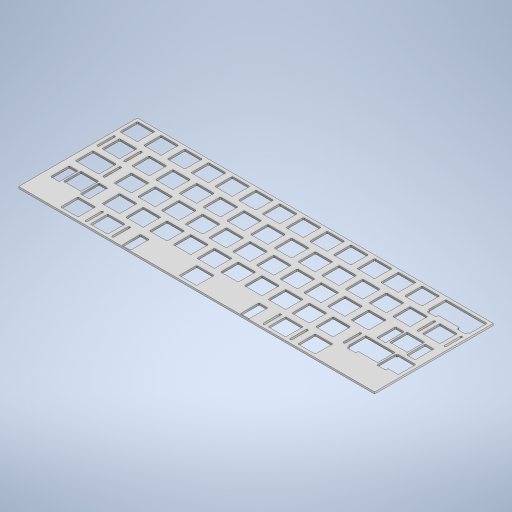
# Autodesk Inventor part: plate
Saved by Autodesk Inventor 2024.2 (Build 282272000, 272)
## iProperties
Created: 2024-07-29
Part Number: plate
Material: Generic
Document SubType Name: Modeling
Designer: Eric
Density: 1 g/cm^3
Appearance: Default
Author: Eric
Autodesk Inventor part; units mm, degrees
ref_plane "YZ Plane" through (0, 0, 0) normal (1, 0, 0) x (0, 1, 0)
ref_plane "XZ Plane" through (0, 0, 0) normal (0, 1, 0) x (-1, 0, 0)
ref_plane "XY Plane" through (0, 0, 0) normal (0, 0, 1) x (1, 0, 0)
sketch "Sketch1" plane through (0, 0, 0) normal (0, 1, 0) x (-1, 0, 0)
  line L0 (-3.025, 2.525) -> (-16.025, 2.525)
  line L1 (-3.025, 16.525) -> (-16.025, 16.525)
  line L2 (-2.525, 3.025) -> (-2.525, 16.025)
  line L3 (-16.525, 3.025) -> (-16.525, 16.025)
  arc A0 (-3.025, 2.525) -> (-2.525, 3.025) centre (-3.025, 3.025) ccw
  arc A1 (-16.525, 3.025) -> (-16.025, 2.525) centre (-16.025, 3.025) ccw
  arc A2 (-2.525, 16.025) -> (-3.025, 16.525) centre (-3.025, 16.025) ccw
  arc A3 (-16.025, 16.525) -> (-16.525, 16.025) centre (-16.025, 16.025) ccw
  line L4 (-22.075, 2.525) -> (-35.075, 2.525)
  line L5 (-22.075, 16.525) -> (-35.075, 16.525)
  line L6 (-21.575, 3.025) -> (-21.575, 16.025)
  line L7 (-35.575, 3.025) -> (-35.575, 16.025)
  arc A4 (-22.075, 2.525) -> (-21.575, 3.025) centre (-22.075, 3.025) ccw
  arc A5 (-35.575, 3.025) -> (-35.075, 2.525) centre (-35.075, 3.025) ccw
  arc A6 (-21.575, 16.025) -> (-22.075, 16.525) centre (-22.075, 16.025) ccw
  arc A7 (-35.075, 16.525) -> (-35.575, 16.025) centre (-35.075, 16.025) ccw
  line L8 (-41.125, 2.525) -> (-54.125, 2.525)
  line L9 (-41.125, 16.525) -> (-54.125, 16.525)
  line L10 (-40.625, 3.025) -> (-40.625, 16.025)
  line L11 (-54.625, 3.025) -> (-54.625, 16.025)
  arc A8 (-41.125, 2.525) -> (-40.625, 3.025) centre (-41.125, 3.025) ccw
  arc A9 (-54.625, 3.025) -> (-54.125, 2.525) centre (-54.125, 3.025) ccw
  arc A10 (-40.625, 16.025) -> (-41.125, 16.525) centre (-41.125, 16.025) ccw
  arc A11 (-54.125, 16.525) -> (-54.625, 16.025) centre (-54.125, 16.025) ccw
  line L12 (-60.175, 2.525) -> (-73.175, 2.525)
  line L13 (-60.175, 16.525) -> (-73.175, 16.525)
  line L14 (-59.675, 3.025) -> (-59.675, 16.025)
  line L15 (-73.675, 3.025) -> (-73.675, 16.025)
  arc A12 (-60.175, 2.525) -> (-59.675, 3.025) centre (-60.175, 3.025) ccw
  arc A13 (-73.675, 3.025) -> (-73.175, 2.525) centre (-73.175, 3.025) ccw
  arc A14 (-59.675, 16.025) -> (-60.175, 16.525) centre (-60.175, 16.025) ccw
  arc A15 (-73.175, 16.525) -> (-73.675, 16.025) centre (-73.175, 16.025) ccw
  line L16 (-79.225, 2.525) -> (-92.225, 2.525)
  line L17 (-79.225, 16.525) -> (-92.225, 16.525)
  line L18 (-78.725, 3.025) -> (-78.725, 16.025)
  line L19 (-92.725, 3.025) -> (-92.725, 16.025)
  arc A16 (-79.225, 2.525) -> (-78.725, 3.025) centre (-79.225, 3.025) ccw
  arc A17 (-92.725, 3.025) -> (-92.225, 2.525) centre (-92.225, 3.025) ccw
  arc A18 (-78.725, 16.025) -> (-79.225, 16.525) centre (-79.225, 16.025) ccw
  arc A19 (-92.225, 16.525) -> (-92.725, 16.025) centre (-92.225, 16.025) ccw
  line L20 (-98.275, 2.525) -> (-111.275, 2.525)
  line L21 (-98.275, 16.525) -> (-111.275, 16.525)
  line L22 (-97.775, 3.025) -> (-97.775, 16.025)
  line L23 (-111.775, 3.025) -> (-111.775, 16.025)
  arc A20 (-98.275, 2.525) -> (-97.775, 3.025) centre (-98.275, 3.025) ccw
  arc A21 (-111.775, 3.025) -> (-111.275, 2.525) centre (-111.275, 3.025) ccw
  arc A22 (-97.775, 16.025) -> (-98.275, 16.525) centre (-98.275, 16.025) ccw
  arc A23 (-111.275, 16.525) -> (-111.775, 16.025) centre (-111.275, 16.025) ccw
  line L24 (-117.325, 2.525) -> (-130.325, 2.525)
  line L25 (-117.325, 16.525) -> (-130.325, 16.525)
  line L26 (-116.825, 3.025) -> (-116.825, 16.025)
  line L27 (-130.825, 3.025) -> (-130.825, 16.025)
  arc A24 (-117.325, 2.525) -> (-116.825, 3.025) centre (-117.325, 3.025) ccw
  arc A25 (-130.825, 3.025) -> (-130.325, 2.525) centre (-130.325, 3.025) ccw
  arc A26 (-116.825, 16.025) -> (-117.325, 16.525) centre (-117.325, 16.025) ccw
  arc A27 (-130.325, 16.525) -> (-130.825, 16.025) centre (-130.325, 16.025) ccw
  line L28 (-136.375, 2.525) -> (-149.375, 2.525)
  line L29 (-136.375, 16.525) -> (-149.375, 16.525)
  line L30 (-135.875, 3.025) -> (-135.875, 16.025)
  line L31 (-149.875, 3.025) -> (-149.875, 16.025)
  arc A28 (-136.375, 2.525) -> (-135.875, 3.025) centre (-136.375, 3.025) ccw
  arc A29 (-149.875, 3.025) -> (-149.375, 2.525) centre (-149.375, 3.025) ccw
  arc A30 (-135.875, 16.025) -> (-136.375, 16.525) centre (-136.375, 16.025) ccw
  arc A31 (-149.375, 16.525) -> (-149.875, 16.025) centre (-149.375, 16.025) ccw
  line L32 (-155.425, 2.525) -> (-168.425, 2.525)
  line L33 (-155.425, 16.525) -> (-168.425, 16.525)
  line L34 (-154.925, 3.025) -> (-154.925, 16.025)
  line L35 (-168.925, 3.025) -> (-168.925, 16.025)
  arc A32 (-155.425, 2.525) -> (-154.925, 3.025) centre (-155.425, 3.025) ccw
  arc A33 (-168.925, 3.025) -> (-168.425, 2.525) centre (-168.425, 3.025) ccw
  arc A34 (-154.925, 16.025) -> (-155.425, 16.525) centre (-155.425, 16.025) ccw
  arc A35 (-168.425, 16.525) -> (-168.925, 16.025) centre (-168.425, 16.025) ccw
  line L36 (-174.475, 2.525) -> (-187.475, 2.525)
  line L37 (-174.475, 16.525) -> (-187.475, 16.525)
  line L38 (-173.975, 3.025) -> (-173.975, 16.025)
  line L39 (-187.975, 3.025) -> (-187.975, 16.025)
  arc A36 (-174.475, 2.525) -> (-173.975, 3.025) centre (-174.475, 3.025) ccw
  arc A37 (-187.975, 3.025) -> (-187.475, 2.525) centre (-187.475, 3.025) ccw
  arc A38 (-173.975, 16.025) -> (-174.475, 16.525) centre (-174.475, 16.025) ccw
  arc A39 (-187.475, 16.525) -> (-187.975, 16.025) centre (-187.475, 16.025) ccw
  line L40 (-193.525, 2.525) -> (-206.525, 2.525)
  line L41 (-193.525, 16.525) -> (-206.525, 16.525)
  line L42 (-193.025, 3.025) -> (-193.025, 16.025)
  line L43 (-207.025, 3.025) -> (-207.025, 16.025)
  arc A40 (-193.525, 2.525) -> (-193.025, 3.025) centre (-193.525, 3.025) ccw
  arc A41 (-207.025, 3.025) -> (-206.525, 2.525) centre (-206.525, 3.025) ccw
  arc A42 (-193.025, 16.025) -> (-193.525, 16.525) centre (-193.525, 16.025) ccw
  arc A43 (-206.525, 16.525) -> (-207.025, 16.025) centre (-206.525, 16.025) ccw
  line L44 (-212.575, 2.525) -> (-225.575, 2.525)
  line L45 (-212.575, 16.525) -> (-225.575, 16.525)
  line L46 (-212.075, 3.025) -> (-212.075, 16.025)
  line L47 (-226.075, 3.025) -> (-226.075, 16.025)
  arc A44 (-212.575, 2.525) -> (-212.075, 3.025) centre (-212.575, 3.025) ccw
  arc A45 (-226.075, 3.025) -> (-225.575, 2.525) centre (-225.575, 3.025) ccw
  arc A46 (-212.075, 16.025) -> (-212.575, 16.525) centre (-212.575, 16.025) ccw
  arc A47 (-225.575, 16.525) -> (-226.075, 16.025) centre (-225.575, 16.025) ccw
  line L48 (-231.625, 2.525) -> (-244.625, 2.525)
  line L49 (-231.625, 16.525) -> (-244.625, 16.525)
  line L50 (-231.125, 3.025) -> (-231.125, 16.025)
  line L51 (-245.125, 3.025) -> (-245.125, 16.025)
  arc A48 (-231.625, 2.525) -> (-231.125, 3.025) centre (-231.625, 3.025) ccw
  arc A49 (-245.125, 3.025) -> (-244.625, 2.525) centre (-244.625, 3.025) ccw
  arc A50 (-231.125, 16.025) -> (-231.625, 16.525) centre (-231.625, 16.025) ccw
  arc A51 (-244.625, 16.525) -> (-245.125, 16.025) centre (-244.625, 16.025) ccw
  line L52 (-260.2, 2.525) -> (-273.2, 2.525)
  line L53 (-260.2, 16.525) -> (-273.2, 16.525)
  line L54 (-251.762, 18.525) -> (-257.762, 18.525)
  line L55 (-251.262, 17.025) -> (-251.262, 18.025)
  line L56 (-258.262, 17.025) -> (-258.262, 18.025)
  arc A52 (-251.262, 18.025) -> (-251.762, 18.525) centre (-251.762, 18.025) ccw
  arc A53 (-257.762, 18.525) -> (-258.262, 18.025) centre (-257.762, 18.025) ccw
  line L57 (-275.638, 18.525) -> (-281.638, 18.525)
  line L58 (-275.138, 17.025) -> (-275.138, 18.025)
  line L59 (-282.138, 17.025) -> (-282.138, 18.025)
  arc A54 (-275.138, 18.025) -> (-275.638, 18.525) centre (-275.638, 18.025) ccw
  arc A55 (-281.638, 18.525) -> (-282.138, 18.025) centre (-281.638, 18.025) ccw
  line L60 (-250.675, 2.525) -> (-263.675, 2.525)
  line L61 (-250.175, 3.025) -> (-250.175, 16.025)
  arc A56 (-250.675, 2.525) -> (-250.175, 3.025) centre (-250.675, 3.025) ccw
  arc A57 (-250.175, 16.025) -> (-250.675, 16.525) centre (-250.675, 16.025) ccw
  line L62 (-269.725, 2.525) -> (-282.725, 2.525)
  line L63 (-283.225, 3.025) -> (-283.225, 16.025)
  arc A58 (-283.225, 3.025) -> (-282.725, 2.525) centre (-282.725, 3.025) ccw
  arc A59 (-282.725, 16.525) -> (-283.225, 16.025) centre (-282.725, 16.025) ccw
  line L64 (-7.7875, 21.575) -> (-20.7875, 21.575)
  line L65 (-7.7875, 35.575) -> (-20.7875, 35.575)
  line L66 (-7.2875, 22.075) -> (-7.2875, 35.075)
  line L67 (-21.2875, 22.075) -> (-21.2875, 35.075)
  arc A60 (-7.7875, 21.575) -> (-7.2875, 22.075) centre (-7.7875, 22.075) ccw
  arc A61 (-21.2875, 22.075) -> (-20.7875, 21.575) centre (-20.7875, 22.075) ccw
  arc A62 (-7.2875, 35.075) -> (-7.7875, 35.575) centre (-7.7875, 35.075) ccw
  arc A63 (-20.7875, 35.575) -> (-21.2875, 35.075) centre (-20.7875, 35.075) ccw
  line L68 (-3.2875, 21.575) -> (-3.7875, 21.575)
  line L69 (-3.2875, 35.575) -> (-3.7875, 35.575)
  line L70 (-2.7875, 22.075) -> (-2.7875, 35.075)
  line L71 (-4.2875, 22.075) -> (-4.2875, 35.075)
  arc A64 (-3.2875, 21.575) -> (-2.7875, 22.075) centre (-3.2875, 22.075) ccw
  arc A65 (-4.2875, 22.075) -> (-3.7875, 21.575) centre (-3.7875, 22.075) ccw
  arc A66 (-2.7875, 35.075) -> (-3.2875, 35.575) centre (-3.2875, 35.075) ccw
  arc A67 (-3.7875, 35.575) -> (-4.2875, 35.075) centre (-3.7875, 35.075) ccw
  line L72 (-24.7875, 21.575) -> (-25.2875, 21.575)
  line L73 (-24.7875, 35.575) -> (-25.2875, 35.575)
  line L74 (-24.2875, 22.075) -> (-24.2875, 35.075)
  line L75 (-25.7875, 22.075) -> (-25.7875, 35.075)
  arc A68 (-24.7875, 21.575) -> (-24.2875, 22.075) centre (-24.7875, 22.075) ccw
  arc A69 (-25.7875, 22.075) -> (-25.2875, 21.575) centre (-25.2875, 22.075) ccw
  arc A70 (-24.2875, 35.075) -> (-24.7875, 35.575) centre (-24.7875, 35.075) ccw
  arc A71 (-25.2875, 35.575) -> (-25.7875, 35.075) centre (-25.2875, 35.075) ccw
  line L76 (-31.6, 21.575) -> (-44.6, 21.575)
  line L77 (-31.6, 35.575) -> (-44.6, 35.575)
  line L78 (-31.1, 22.075) -> (-31.1, 35.075)
  line L79 (-45.1, 22.075) -> (-45.1, 35.075)
  arc A72 (-31.6, 21.575) -> (-31.1, 22.075) centre (-31.6, 22.075) ccw
  arc A73 (-45.1, 22.075) -> (-44.6, 21.575) centre (-44.6, 22.075) ccw
  arc A74 (-31.1, 35.075) -> (-31.6, 35.575) centre (-31.6, 35.075) ccw
  arc A75 (-44.6, 35.575) -> (-45.1, 35.075) centre (-44.6, 35.075) ccw
  line L80 (-50.65, 21.575) -> (-63.65, 21.575)
  line L81 (-50.65, 35.575) -> (-63.65, 35.575)
  line L82 (-50.15, 22.075) -> (-50.15, 35.075)
  line L83 (-64.15, 22.075) -> (-64.15, 35.075)
  arc A76 (-50.65, 21.575) -> (-50.15, 22.075) centre (-50.65, 22.075) ccw
  arc A77 (-64.15, 22.075) -> (-63.65, 21.575) centre (-63.65, 22.075) ccw
  arc A78 (-50.15, 35.075) -> (-50.65, 35.575) centre (-50.65, 35.075) ccw
  arc A79 (-63.65, 35.575) -> (-64.15, 35.075) centre (-63.65, 35.075) ccw
  line L84 (-69.7, 21.575) -> (-82.7, 21.575)
  line L85 (-69.7, 35.575) -> (-82.7, 35.575)
  line L86 (-69.2, 22.075) -> (-69.2, 35.075)
  line L87 (-83.2, 22.075) -> (-83.2, 35.075)
  arc A80 (-69.7, 21.575) -> (-69.2, 22.075) centre (-69.7, 22.075) ccw
  arc A81 (-83.2, 22.075) -> (-82.7, 21.575) centre (-82.7, 22.075) ccw
  arc A82 (-69.2, 35.075) -> (-69.7, 35.575) centre (-69.7, 35.075) ccw
  arc A83 (-82.7, 35.575) -> (-83.2, 35.075) centre (-82.7, 35.075) ccw
  line L88 (-88.75, 21.575) -> (-101.75, 21.575)
  line L89 (-88.75, 35.575) -> (-101.75, 35.575)
  line L90 (-88.25, 22.075) -> (-88.25, 35.075)
  line L91 (-102.25, 22.075) -> (-102.25, 35.075)
  arc A84 (-88.75, 21.575) -> (-88.25, 22.075) centre (-88.75, 22.075) ccw
  arc A85 (-102.25, 22.075) -> (-101.75, 21.575) centre (-101.75, 22.075) ccw
  arc A86 (-88.25, 35.075) -> (-88.75, 35.575) centre (-88.75, 35.075) ccw
  arc A87 (-101.75, 35.575) -> (-102.25, 35.075) centre (-101.75, 35.075) ccw
  line L92 (-107.8, 21.575) -> (-120.8, 21.575)
  line L93 (-107.8, 35.575) -> (-120.8, 35.575)
  line L94 (-107.3, 22.075) -> (-107.3, 35.075)
  line L95 (-121.3, 22.075) -> (-121.3, 35.075)
  arc A88 (-107.8, 21.575) -> (-107.3, 22.075) centre (-107.8, 22.075) ccw
  arc A89 (-121.3, 22.075) -> (-120.8, 21.575) centre (-120.8, 22.075) ccw
  arc A90 (-107.3, 35.075) -> (-107.8, 35.575) centre (-107.8, 35.075) ccw
  arc A91 (-120.8, 35.575) -> (-121.3, 35.075) centre (-120.8, 35.075) ccw
  line L96 (-126.85, 21.575) -> (-139.85, 21.575)
  line L97 (-126.85, 35.575) -> (-139.85, 35.575)
  line L98 (-126.35, 22.075) -> (-126.35, 35.075)
  line L99 (-140.35, 22.075) -> (-140.35, 35.075)
  arc A92 (-126.85, 21.575) -> (-126.35, 22.075) centre (-126.85, 22.075) ccw
  arc A93 (-140.35, 22.075) -> (-139.85, 21.575) centre (-139.85, 22.075) ccw
  arc A94 (-126.35, 35.075) -> (-126.85, 35.575) centre (-126.85, 35.075) ccw
  arc A95 (-139.85, 35.575) -> (-140.35, 35.075) centre (-139.85, 35.075) ccw
  line L100 (-145.9, 21.575) -> (-158.9, 21.575)
  line L101 (-145.9, 35.575) -> (-158.9, 35.575)
  line L102 (-145.4, 22.075) -> (-145.4, 35.075)
  line L103 (-159.4, 22.075) -> (-159.4, 35.075)
  arc A96 (-145.9, 21.575) -> (-145.4, 22.075) centre (-145.9, 22.075) ccw
  arc A97 (-159.4, 22.075) -> (-158.9, 21.575) centre (-158.9, 22.075) ccw
  arc A98 (-145.4, 35.075) -> (-145.9, 35.575) centre (-145.9, 35.075) ccw
  arc A99 (-158.9, 35.575) -> (-159.4, 35.075) centre (-158.9, 35.075) ccw
  line L104 (-164.95, 21.575) -> (-177.95, 21.575)
  line L105 (-164.95, 35.575) -> (-177.95, 35.575)
  line L106 (-164.45, 22.075) -> (-164.45, 35.075)
  line L107 (-178.45, 22.075) -> (-178.45, 35.075)
  arc A100 (-164.95, 21.575) -> (-164.45, 22.075) centre (-164.95, 22.075) ccw
  arc A101 (-178.45, 22.075) -> (-177.95, 21.575) centre (-177.95, 22.075) ccw
  arc A102 (-164.45, 35.075) -> (-164.95, 35.575) centre (-164.95, 35.075) ccw
  arc A103 (-177.95, 35.575) -> (-178.45, 35.075) centre (-177.95, 35.075) ccw
  line L108 (-184, 21.575) -> (-197, 21.575)
  line L109 (-184, 35.575) -> (-197, 35.575)
  line L110 (-183.5, 22.075) -> (-183.5, 35.075)
  line L111 (-197.5, 22.075) -> (-197.5, 35.075)
  arc A104 (-184, 21.575) -> (-183.5, 22.075) centre (-184, 22.075) ccw
  arc A105 (-197.5, 22.075) -> (-197, 21.575) centre (-197, 22.075) ccw
  arc A106 (-183.5, 35.075) -> (-184, 35.575) centre (-184, 35.075) ccw
  arc A107 (-197, 35.575) -> (-197.5, 35.075) centre (-197, 35.075) ccw
  line L112 (-203.05, 21.575) -> (-216.05, 21.575)
  line L113 (-203.05, 35.575) -> (-216.05, 35.575)
  line L114 (-202.55, 22.075) -> (-202.55, 35.075)
  line L115 (-216.55, 22.075) -> (-216.55, 35.075)
  arc A108 (-203.05, 21.575) -> (-202.55, 22.075) centre (-203.05, 22.075) ccw
  arc A109 (-216.55, 22.075) -> (-216.05, 21.575) centre (-216.05, 22.075) ccw
  arc A110 (-202.55, 35.075) -> (-203.05, 35.575) centre (-203.05, 35.075) ccw
  arc A111 (-216.05, 35.575) -> (-216.55, 35.075) centre (-216.05, 35.075) ccw
  line L116 (-222.1, 21.575) -> (-235.1, 21.575)
  line L117 (-222.1, 35.575) -> (-235.1, 35.575)
  line L118 (-221.6, 22.075) -> (-221.6, 35.075)
  line L119 (-235.6, 22.075) -> (-235.6, 35.075)
  arc A112 (-222.1, 21.575) -> (-221.6, 22.075) centre (-222.1, 22.075) ccw
  arc A113 (-235.6, 22.075) -> (-235.1, 21.575) centre (-235.1, 22.075) ccw
  arc A114 (-221.6, 35.075) -> (-222.1, 35.575) centre (-222.1, 35.075) ccw
  arc A115 (-235.1, 35.575) -> (-235.6, 35.075) centre (-235.1, 35.075) ccw
  line L120 (-241.15, 21.575) -> (-254.15, 21.575)
  line L121 (-241.15, 35.575) -> (-254.15, 35.575)
  line L122 (-240.65, 22.075) -> (-240.65, 35.075)
  line L123 (-254.65, 22.075) -> (-254.65, 35.075)
  arc A116 (-241.15, 21.575) -> (-240.65, 22.075) centre (-241.15, 22.075) ccw
  arc A117 (-254.65, 22.075) -> (-254.15, 21.575) centre (-254.15, 22.075) ccw
  arc A118 (-240.65, 35.075) -> (-241.15, 35.575) centre (-241.15, 35.075) ccw
  arc A119 (-254.15, 35.575) -> (-254.65, 35.075) centre (-254.15, 35.075) ccw
  line L124 (-264.9625, 21.575) -> (-277.9625, 21.575)
  line L125 (-264.9625, 35.575) -> (-277.9625, 35.575)
  line L126 (-264.4625, 22.075) -> (-264.4625, 35.075)
  line L127 (-278.4625, 22.075) -> (-278.4625, 35.075)
  arc A120 (-264.9625, 21.575) -> (-264.4625, 22.075) centre (-264.9625, 22.075) ccw
  arc A121 (-278.4625, 22.075) -> (-277.9625, 21.575) centre (-277.9625, 22.075) ccw
  arc A122 (-264.4625, 35.075) -> (-264.9625, 35.575) centre (-264.9625, 35.075) ccw
  arc A123 (-277.9625, 35.575) -> (-278.4625, 35.075) centre (-277.9625, 35.075) ccw
  line L128 (-260.4625, 21.575) -> (-260.9625, 21.575)
  line L129 (-260.4625, 35.575) -> (-260.9625, 35.575)
  line L130 (-259.9625, 22.075) -> (-259.9625, 35.075)
  line L131 (-261.4625, 22.075) -> (-261.4625, 35.075)
  arc A124 (-260.4625, 21.575) -> (-259.9625, 22.075) centre (-260.4625, 22.075) ccw
  arc A125 (-261.4625, 22.075) -> (-260.9625, 21.575) centre (-260.9625, 22.075) ccw
  arc A126 (-259.9625, 35.075) -> (-260.4625, 35.575) centre (-260.4625, 35.075) ccw
  arc A127 (-260.9625, 35.575) -> (-261.4625, 35.075) centre (-260.9625, 35.075) ccw
  line L132 (-281.9625, 21.575) -> (-282.4625, 21.575)
  line L133 (-281.9625, 35.575) -> (-282.4625, 35.575)
  line L134 (-281.4625, 22.075) -> (-281.4625, 35.075)
  line L135 (-282.9625, 22.075) -> (-282.9625, 35.075)
  arc A128 (-281.9625, 21.575) -> (-281.4625, 22.075) centre (-281.9625, 22.075) ccw
  arc A129 (-282.9625, 22.075) -> (-282.4625, 21.575) centre (-282.4625, 22.075) ccw
  arc A130 (-281.4625, 35.075) -> (-281.9625, 35.575) centre (-281.9625, 35.075) ccw
  arc A131 (-282.4625, 35.575) -> (-282.9625, 35.075) centre (-282.4625, 35.075) ccw
  line L136 (-10.1687, 40.625) -> (-23.1687, 40.625)
  line L137 (-10.1687, 54.625) -> (-23.1687, 54.625)
  line L138 (-23.6687, 41.125) -> (-23.6687, 54.125)
  arc A132 (-23.6687, 41.125) -> (-23.1687, 40.625) centre (-23.1687, 41.125) ccw
  arc A133 (-23.1687, 54.625) -> (-23.6687, 54.125) centre (-23.1687, 54.125) ccw
  line L139 (-5.6687, 40.625) -> (-6.1687, 40.625)
  line L140 (-5.6687, 54.625) -> (-6.1687, 54.625)
  line L141 (-27.1687, 40.625) -> (-27.6687, 40.625)
  line L142 (-27.1687, 54.625) -> (-27.6687, 54.625)
  line L143 (-26.6687, 41.125) -> (-26.6687, 54.125)
  line L144 (-28.1687, 41.125) -> (-28.1687, 54.125)
  arc A134 (-27.1687, 40.625) -> (-26.6687, 41.125) centre (-27.1687, 41.125) ccw
  arc A135 (-28.1687, 41.125) -> (-27.6687, 40.625) centre (-27.6687, 41.125) ccw
  arc A136 (-26.6688, 54.125) -> (-27.1687, 54.625) centre (-27.1687, 54.125) ccw
  arc A137 (-27.6687, 54.625) -> (-28.1687, 54.125) centre (-27.6688, 54.125) ccw
  line L145 (-5.4062, 40.625) -> (-18.4062, 40.625)
  line L146 (-5.4062, 54.625) -> (-18.4062, 54.625)
  line L147 (-4.9062, 41.125) -> (-4.9062, 54.125)
  arc A138 (-5.4062, 40.625) -> (-4.9062, 41.125) centre (-5.4062, 41.125) ccw
  arc A139 (-4.9062, 54.125) -> (-5.4062, 54.625) centre (-5.4062, 54.125) ccw
  line L148 (-36.3625, 40.625) -> (-49.3625, 40.625)
  line L149 (-36.3625, 54.625) -> (-49.3625, 54.625)
  line L150 (-35.8625, 41.125) -> (-35.8625, 54.125)
  line L151 (-49.8625, 41.125) -> (-49.8625, 54.125)
  arc A140 (-36.3625, 40.625) -> (-35.8625, 41.125) centre (-36.3625, 41.125) ccw
  arc A141 (-49.8625, 41.125) -> (-49.3625, 40.625) centre (-49.3625, 41.125) ccw
  arc A142 (-35.8625, 54.125) -> (-36.3625, 54.625) centre (-36.3625, 54.125) ccw
  arc A143 (-49.3625, 54.625) -> (-49.8625, 54.125) centre (-49.3625, 54.125) ccw
  line L152 (-55.4125, 40.625) -> (-68.4125, 40.625)
  line L153 (-55.4125, 54.625) -> (-68.4125, 54.625)
  line L154 (-54.9125, 41.125) -> (-54.9125, 54.125)
  line L155 (-68.9125, 41.125) -> (-68.9125, 54.125)
  arc A144 (-55.4125, 40.625) -> (-54.9125, 41.125) centre (-55.4125, 41.125) ccw
  arc A145 (-68.9125, 41.125) -> (-68.4125, 40.625) centre (-68.4125, 41.125) ccw
  arc A146 (-54.9125, 54.125) -> (-55.4125, 54.625) centre (-55.4125, 54.125) ccw
  arc A147 (-68.4125, 54.625) -> (-68.9125, 54.125) centre (-68.4125, 54.125) ccw
  line L156 (-74.4625, 40.625) -> (-87.4625, 40.625)
  line L157 (-74.4625, 54.625) -> (-87.4625, 54.625)
  line L158 (-73.9625, 41.125) -> (-73.9625, 54.125)
  line L159 (-87.9625, 41.125) -> (-87.9625, 54.125)
  arc A148 (-74.4625, 40.625) -> (-73.9625, 41.125) centre (-74.4625, 41.125) ccw
  arc A149 (-87.9625, 41.125) -> (-87.4625, 40.625) centre (-87.4625, 41.125) ccw
  arc A150 (-73.9625, 54.125) -> (-74.4625, 54.625) centre (-74.4625, 54.125) ccw
  arc A151 (-87.4625, 54.625) -> (-87.9625, 54.125) centre (-87.4625, 54.125) ccw
  line L160 (-93.5125, 40.625) -> (-106.5125, 40.625)
  line L161 (-93.5125, 54.625) -> (-106.5125, 54.625)
  line L162 (-93.0125, 41.125) -> (-93.0125, 54.125)
  line L163 (-107.0125, 41.125) -> (-107.0125, 54.125)
  arc A152 (-93.5125, 40.625) -> (-93.0125, 41.125) centre (-93.5125, 41.125) ccw
  arc A153 (-107.0125, 41.125) -> (-106.5125, 40.625) centre (-106.5125, 41.125) ccw
  arc A154 (-93.0125, 54.125) -> (-93.5125, 54.625) centre (-93.5125, 54.125) ccw
  arc A155 (-106.5125, 54.625) -> (-107.0125, 54.125) centre (-106.5125, 54.125) ccw
  line L164 (-112.5625, 40.625) -> (-125.5625, 40.625)
  line L165 (-112.5625, 54.625) -> (-125.5625, 54.625)
  line L166 (-112.0625, 41.125) -> (-112.0625, 54.125)
  line L167 (-126.0625, 41.125) -> (-126.0625, 54.125)
  arc A156 (-112.5625, 40.625) -> (-112.0625, 41.125) centre (-112.5625, 41.125) ccw
  arc A157 (-126.0625, 41.125) -> (-125.5625, 40.625) centre (-125.5625, 41.125) ccw
  arc A158 (-112.0625, 54.125) -> (-112.5625, 54.625) centre (-112.5625, 54.125) ccw
  arc A159 (-125.5625, 54.625) -> (-126.0625, 54.125) centre (-125.5625, 54.125) ccw
  line L168 (-131.6125, 40.625) -> (-144.6125, 40.625)
  line L169 (-131.6125, 54.625) -> (-144.6125, 54.625)
  line L170 (-131.1125, 41.125) -> (-131.1125, 54.125)
  line L171 (-145.1125, 41.125) -> (-145.1125, 54.125)
  arc A160 (-131.6125, 40.625) -> (-131.1125, 41.125) centre (-131.6125, 41.125) ccw
  arc A161 (-145.1125, 41.125) -> (-144.6125, 40.625) centre (-144.6125, 41.125) ccw
  arc A162 (-131.1125, 54.125) -> (-131.6125, 54.625) centre (-131.6125, 54.125) ccw
  arc A163 (-144.6125, 54.625) -> (-145.1125, 54.125) centre (-144.6125, 54.125) ccw
  line L172 (-150.6625, 40.625) -> (-163.6625, 40.625)
  line L173 (-150.6625, 54.625) -> (-163.6625, 54.625)
  line L174 (-150.1625, 41.125) -> (-150.1625, 54.125)
  line L175 (-164.1625, 41.125) -> (-164.1625, 54.125)
  arc A164 (-150.6625, 40.625) -> (-150.1625, 41.125) centre (-150.6625, 41.125) ccw
  arc A165 (-164.1625, 41.125) -> (-163.6625, 40.625) centre (-163.6625, 41.125) ccw
  arc A166 (-150.1625, 54.125) -> (-150.6625, 54.625) centre (-150.6625, 54.125) ccw
  arc A167 (-163.6625, 54.625) -> (-164.1625, 54.125) centre (-163.6625, 54.125) ccw
  line L176 (-169.7125, 40.625) -> (-182.7125, 40.625)
  line L177 (-169.7125, 54.625) -> (-182.7125, 54.625)
  line L178 (-169.2125, 41.125) -> (-169.2125, 54.125)
  line L179 (-183.2125, 41.125) -> (-183.2125, 54.125)
  arc A168 (-169.7125, 40.625) -> (-169.2125, 41.125) centre (-169.7125, 41.125) ccw
  arc A169 (-183.2125, 41.125) -> (-182.7125, 40.625) centre (-182.7125, 41.125) ccw
  arc A170 (-169.2125, 54.125) -> (-169.7125, 54.625) centre (-169.7125, 54.125) ccw
  arc A171 (-182.7125, 54.625) -> (-183.2125, 54.125) centre (-182.7125, 54.125) ccw
  line L180 (-188.7625, 40.625) -> (-201.7625, 40.625)
  line L181 (-188.7625, 54.625) -> (-201.7625, 54.625)
  line L182 (-188.2625, 41.125) -> (-188.2625, 54.125)
  line L183 (-202.2625, 41.125) -> (-202.2625, 54.125)
  arc A172 (-188.7625, 40.625) -> (-188.2625, 41.125) centre (-188.7625, 41.125) ccw
  arc A173 (-202.2625, 41.125) -> (-201.7625, 40.625) centre (-201.7625, 41.125) ccw
  arc A174 (-188.2625, 54.125) -> (-188.7625, 54.625) centre (-188.7625, 54.125) ccw
  arc A175 (-201.7625, 54.625) -> (-202.2625, 54.125) centre (-201.7625, 54.125) ccw
  line L184 (-207.8125, 40.625) -> (-220.8125, 40.625)
  line L185 (-207.8125, 54.625) -> (-220.8125, 54.625)
  line L186 (-207.3125, 41.125) -> (-207.3125, 54.125)
  line L187 (-221.3125, 41.125) -> (-221.3125, 54.125)
  arc A176 (-207.8125, 40.625) -> (-207.3125, 41.125) centre (-207.8125, 41.125) ccw
  arc A177 (-221.3125, 41.125) -> (-220.8125, 40.625) centre (-220.8125, 41.125) ccw
  arc A178 (-207.3125, 54.125) -> (-207.8125, 54.625) centre (-207.8125, 54.125) ccw
  arc A179 (-220.8125, 54.625) -> (-221.3125, 54.125) centre (-220.8125, 54.125) ccw
  line L188 (-226.8625, 40.625) -> (-239.8625, 40.625)
  line L189 (-226.8625, 54.625) -> (-239.8625, 54.625)
  line L190 (-226.3625, 41.125) -> (-226.3625, 54.125)
  line L191 (-240.3625, 41.125) -> (-240.3625, 54.125)
  arc A180 (-226.8625, 40.625) -> (-226.3625, 41.125) centre (-226.8625, 41.125) ccw
  arc A181 (-240.3625, 41.125) -> (-239.8625, 40.625) centre (-239.8625, 41.125) ccw
  arc A182 (-226.3625, 54.125) -> (-226.8625, 54.625) centre (-226.8625, 54.125) ccw
  arc A183 (-239.8625, 54.625) -> (-240.3625, 54.125) centre (-239.8625, 54.125) ccw
  line L192 (-257.8188, 40.625) -> (-270.8188, 40.625)
  line L193 (-257.8188, 54.625) -> (-270.8188, 54.625)
  line L194 (-257.3188, 41.125) -> (-257.3187, 54.125)
  line L195 (-271.3188, 41.125) -> (-271.3188, 54.125)
  arc A184 (-257.8188, 40.625) -> (-257.3188, 41.125) centre (-257.8188, 41.125) ccw
  arc A185 (-271.3188, 41.125) -> (-270.8188, 40.625) centre (-270.8188, 41.125) ccw
  arc A186 (-257.3187, 54.125) -> (-257.8188, 54.625) centre (-257.8188, 54.125) ccw
  arc A187 (-270.8188, 54.625) -> (-271.3187, 54.125) centre (-270.8188, 54.125) ccw
  line L196 (-249.3808, 41.625) -> (-255.3808, 41.625)
  line L197 (-249.3807, 56.625) -> (-255.3807, 56.625)
  line L198 (-248.8808, 42.125) -> (-248.8808, 56.125)
  line L199 (-255.8808, 42.125) -> (-255.8808, 56.125)
  arc A188 (-249.3808, 41.625) -> (-248.8808, 42.125) centre (-249.3808, 42.125) ccw
  arc A189 (-255.8807, 42.125) -> (-255.3808, 41.625) centre (-255.3807, 42.125) ccw
  arc A190 (-248.8808, 56.125) -> (-249.3807, 56.625) centre (-249.3808, 56.125) ccw
  arc A191 (-255.3807, 56.625) -> (-255.8808, 56.125) centre (-255.3808, 56.125) ccw
  line L200 (-273.2568, 41.625) -> (-279.2568, 41.625)
  line L201 (-273.2568, 56.625) -> (-279.2568, 56.625)
  line L202 (-272.7568, 42.125) -> (-272.7568, 56.125)
  line L203 (-279.7568, 42.125) -> (-279.7568, 56.125)
  arc A192 (-273.2568, 41.625) -> (-272.7568, 42.125) centre (-273.2568, 42.125) ccw
  arc A193 (-279.7568, 42.125) -> (-279.2568, 41.625) centre (-279.2568, 42.125) ccw
  arc A194 (-272.7568, 56.125) -> (-273.2568, 56.625) centre (-273.2567, 56.125) ccw
  arc A195 (-279.2568, 56.625) -> (-279.7568, 56.125) centre (-279.2568, 56.125) ccw
  line L204 (-14.9312, 59.675) -> (-27.9312, 59.675)
  line L205 (-14.9312, 73.675) -> (-27.9312, 73.675)
  line L206 (-14.4312, 60.175) -> (-14.4312, 73.175)
  line L207 (-28.4312, 60.175) -> (-28.4313, 73.175)
  arc A196 (-14.9312, 59.675) -> (-14.4312, 60.175) centre (-14.9312, 60.175) ccw
  arc A197 (-28.4312, 60.175) -> (-27.9312, 59.675) centre (-27.9312, 60.175) ccw
  arc A198 (-14.4312, 73.175) -> (-14.9312, 73.675) centre (-14.9312, 73.175) ccw
  arc A199 (-27.9312, 73.675) -> (-28.4312, 73.175) centre (-27.9312, 73.175) ccw
  line L208 (-6.4932, 60.675) -> (-12.4932, 60.675)
  line L209 (-6.4932, 75.675) -> (-12.4932, 75.675)
  line L210 (-5.9932, 61.175) -> (-5.9932, 75.175)
  line L211 (-12.9932, 61.175) -> (-12.9932, 75.175)
  arc A200 (-6.4932, 60.675) -> (-5.9932, 61.175) centre (-6.4932, 61.175) ccw
  arc A201 (-12.9932, 61.175) -> (-12.4932, 60.675) centre (-12.4932, 61.175) ccw
  arc A202 (-5.9932, 75.175) -> (-6.4932, 75.675) centre (-6.4932, 75.175) ccw
  arc A203 (-12.4932, 75.675) -> (-12.9932, 75.175) centre (-12.4932, 75.175) ccw
  line L212 (-30.3692, 60.675) -> (-36.3692, 60.675)
  line L213 (-30.3692, 75.675) -> (-36.3692, 75.675)
  line L214 (-29.8693, 61.175) -> (-29.8692, 75.175)
  line L215 (-36.8692, 61.175) -> (-36.8693, 75.175)
  arc A204 (-30.3692, 60.675) -> (-29.8693, 61.175) centre (-30.3693, 61.175) ccw
  arc A205 (-36.8692, 61.175) -> (-36.3692, 60.675) centre (-36.3692, 61.175) ccw
  arc A206 (-29.8692, 75.175) -> (-30.3692, 75.675) centre (-30.3692, 75.175) ccw
  arc A207 (-36.3692, 75.675) -> (-36.8693, 75.175) centre (-36.3693, 75.175) ccw
  line L216 (-45.8875, 59.675) -> (-58.8875, 59.675)
  line L217 (-45.8875, 73.675) -> (-58.8875, 73.675)
  line L218 (-45.3875, 60.175) -> (-45.3875, 73.175)
  line L219 (-59.3875, 60.175) -> (-59.3875, 73.175)
  arc A208 (-45.8875, 59.675) -> (-45.3875, 60.175) centre (-45.8875, 60.175) ccw
  arc A209 (-59.3875, 60.175) -> (-58.8875, 59.675) centre (-58.8875, 60.175) ccw
  arc A210 (-45.3875, 73.175) -> (-45.8875, 73.675) centre (-45.8875, 73.175) ccw
  arc A211 (-58.8875, 73.675) -> (-59.3875, 73.175) centre (-58.8875, 73.175) ccw
  line L220 (-64.9375, 59.675) -> (-77.9375, 59.675)
  line L221 (-64.9375, 73.675) -> (-77.9375, 73.675)
  line L222 (-64.4375, 60.175) -> (-64.4375, 73.175)
  line L223 (-78.4375, 60.175) -> (-78.4375, 73.175)
  arc A212 (-64.9375, 59.675) -> (-64.4375, 60.175) centre (-64.9375, 60.175) ccw
  arc A213 (-78.4375, 60.175) -> (-77.9375, 59.675) centre (-77.9375, 60.175) ccw
  arc A214 (-64.4375, 73.175) -> (-64.9375, 73.675) centre (-64.9375, 73.175) ccw
  arc A215 (-77.9375, 73.675) -> (-78.4375, 73.175) centre (-77.9375, 73.175) ccw
  line L224 (-83.9875, 59.675) -> (-96.9875, 59.675)
  line L225 (-83.9875, 73.675) -> (-96.9875, 73.675)
  line L226 (-83.4875, 60.175) -> (-83.4875, 73.175)
  line L227 (-97.4875, 60.175) -> (-97.4875, 73.175)
  arc A216 (-83.9875, 59.675) -> (-83.4875, 60.175) centre (-83.9875, 60.175) ccw
  arc A217 (-97.4875, 60.175) -> (-96.9875, 59.675) centre (-96.9875, 60.175) ccw
  arc A218 (-83.4875, 73.175) -> (-83.9875, 73.675) centre (-83.9875, 73.175) ccw
  arc A219 (-96.9875, 73.675) -> (-97.4875, 73.175) centre (-96.9875, 73.175) ccw
  line L228 (-103.0375, 59.675) -> (-116.0375, 59.675)
  line L229 (-103.0375, 73.675) -> (-116.0375, 73.675)
  line L230 (-102.5375, 60.175) -> (-102.5375, 73.175)
  line L231 (-116.5375, 60.175) -> (-116.5375, 73.175)
  arc A220 (-103.0375, 59.675) -> (-102.5375, 60.175) centre (-103.0375, 60.175) ccw
  arc A221 (-116.5375, 60.175) -> (-116.0375, 59.675) centre (-116.0375, 60.175) ccw
  arc A222 (-102.5375, 73.175) -> (-103.0375, 73.675) centre (-103.0375, 73.175) ccw
  arc A223 (-116.0375, 73.675) -> (-116.5375, 73.175) centre (-116.0375, 73.175) ccw
  line L232 (-122.0875, 59.675) -> (-135.0875, 59.675)
  line L233 (-122.0875, 73.675) -> (-135.0875, 73.675)
  line L234 (-121.5875, 60.175) -> (-121.5875, 73.175)
  line L235 (-135.5875, 60.175) -> (-135.5875, 73.175)
  arc A224 (-122.0875, 59.675) -> (-121.5875, 60.175) centre (-122.0875, 60.175) ccw
  arc A225 (-135.5875, 60.175) -> (-135.0875, 59.675) centre (-135.0875, 60.175) ccw
  arc A226 (-121.5875, 73.175) -> (-122.0875, 73.675) centre (-122.0875, 73.175) ccw
  arc A227 (-135.0875, 73.675) -> (-135.5875, 73.175) centre (-135.0875, 73.175) ccw
  line L236 (-141.1375, 59.675) -> (-154.1375, 59.675)
  line L237 (-141.1375, 73.675) -> (-154.1375, 73.675)
  line L238 (-140.6375, 60.175) -> (-140.6375, 73.175)
  line L239 (-154.6375, 60.175) -> (-154.6375, 73.175)
  arc A228 (-141.1375, 59.675) -> (-140.6375, 60.175) centre (-141.1375, 60.175) ccw
  arc A229 (-154.6375, 60.175) -> (-154.1375, 59.675) centre (-154.1375, 60.175) ccw
  arc A230 (-140.6375, 73.175) -> (-141.1375, 73.675) centre (-141.1375, 73.175) ccw
  arc A231 (-154.1375, 73.675) -> (-154.6375, 73.175) centre (-154.1375, 73.175) ccw
  line L240 (-160.1875, 59.675) -> (-173.1875, 59.675)
  line L241 (-160.1875, 73.675) -> (-173.1875, 73.675)
  line L242 (-159.6875, 60.175) -> (-159.6875, 73.175)
  line L243 (-173.6875, 60.175) -> (-173.6875, 73.175)
  arc A232 (-160.1875, 59.675) -> (-159.6875, 60.175) centre (-160.1875, 60.175) ccw
  arc A233 (-173.6875, 60.175) -> (-173.1875, 59.675) centre (-173.1875, 60.175) ccw
  arc A234 (-159.6875, 73.175) -> (-160.1875, 73.675) centre (-160.1875, 73.175) ccw
  arc A235 (-173.1875, 73.675) -> (-173.6875, 73.175) centre (-173.1875, 73.175) ccw
  line L244 (-179.2375, 59.675) -> (-192.2375, 59.675)
  line L245 (-179.2375, 73.675) -> (-192.2375, 73.675)
  line L246 (-178.7375, 60.175) -> (-178.7375, 73.175)
  line L247 (-192.7375, 60.175) -> (-192.7375, 73.175)
  arc A236 (-179.2375, 59.675) -> (-178.7375, 60.175) centre (-179.2375, 60.175) ccw
  arc A237 (-192.7375, 60.175) -> (-192.2375, 59.675) centre (-192.2375, 60.175) ccw
  arc A238 (-178.7375, 73.175) -> (-179.2375, 73.675) centre (-179.2375, 73.175) ccw
  arc A239 (-192.2375, 73.675) -> (-192.7375, 73.175) centre (-192.2375, 73.175) ccw
  line L248 (-198.2875, 59.675) -> (-211.2875, 59.675)
  line L249 (-198.2875, 73.675) -> (-211.2875, 73.675)
  line L250 (-197.7875, 60.175) -> (-197.7875, 73.175)
  line L251 (-211.7875, 60.175) -> (-211.7875, 73.175)
  arc A240 (-198.2875, 59.675) -> (-197.7875, 60.175) centre (-198.2875, 60.175) ccw
  arc A241 (-211.7875, 60.175) -> (-211.2875, 59.675) centre (-211.2875, 60.175) ccw
  arc A242 (-197.7875, 73.175) -> (-198.2875, 73.675) centre (-198.2875, 73.175) ccw
  arc A243 (-211.2875, 73.675) -> (-211.7875, 73.175) centre (-211.2875, 73.175) ccw
  line L252 (-217.3375, 59.675) -> (-230.3375, 59.675)
  line L253 (-217.3375, 73.675) -> (-230.3375, 73.675)
  line L254 (-216.8375, 60.175) -> (-216.8375, 73.175)
  line L255 (-230.8375, 60.175) -> (-230.8375, 73.175)
  arc A244 (-217.3375, 59.675) -> (-216.8375, 60.175) centre (-217.3375, 60.175) ccw
  arc A245 (-230.8375, 60.175) -> (-230.3375, 59.675) centre (-230.3375, 60.175) ccw
  arc A246 (-216.8375, 73.175) -> (-217.3375, 73.675) centre (-217.3375, 73.175) ccw
  arc A247 (-230.3375, 73.675) -> (-230.8375, 73.175) centre (-230.3375, 73.175) ccw
  line L256 (-253.0563, 59.675) -> (-266.0563, 59.675)
  line L257 (-253.0563, 73.675) -> (-266.0562, 73.675)
  line L258 (-266.5562, 60.175) -> (-266.5562, 73.175)
  arc A248 (-266.5562, 60.175) -> (-266.0563, 59.675) centre (-266.0563, 60.175) ccw
  arc A249 (-266.0562, 73.675) -> (-266.5562, 73.175) centre (-266.0562, 73.175) ccw
  line L259 (-244.6183, 75.675) -> (-250.6182, 75.675)
  line L260 (-244.1182, 74.175) -> (-244.1182, 75.175)
  line L261 (-251.1182, 74.175) -> (-251.1182, 75.175)
  arc A250 (-244.1182, 75.175) -> (-244.6183, 75.675) centre (-244.6183, 75.175) ccw
  arc A251 (-250.6182, 75.675) -> (-251.1182, 75.175) centre (-250.6182, 75.175) ccw
  line L262 (-268.4943, 60.675) -> (-268.725, 60.675)
  line L263 (-268.4943, 75.675) -> (-274.4943, 75.675)
  line L264 (-267.9942, 61.175) -> (-267.9942, 75.175)
  line L265 (-274.9942, 74.175) -> (-274.9942, 75.175)
  arc A252 (-268.4943, 60.675) -> (-267.9942, 61.175) centre (-268.4943, 61.175) ccw
  arc A253 (-267.9942, 75.175) -> (-268.4942, 75.675) centre (-268.4943, 75.175) ccw
  arc A254 (-274.4943, 75.675) -> (-274.9942, 75.175) centre (-274.4942, 75.175) ccw
  line L266 (-243.5313, 59.675) -> (-256.5313, 59.675)
  line L267 (-243.0312, 60.175) -> (-243.0313, 73.175)
  arc A255 (-243.5313, 59.675) -> (-243.0313, 60.175) centre (-243.5313, 60.175) ccw
  arc A256 (-243.0313, 73.175) -> (-243.5313, 73.675) centre (-243.5313, 73.175) ccw
  line L268 (-239.0313, 59.675) -> (-239.5312, 59.675)
  line L269 (-239.0313, 73.675) -> (-239.5312, 73.675)
  line L270 (-238.5313, 60.175) -> (-238.5312, 73.175)
  line L271 (-240.0312, 60.175) -> (-240.0312, 73.175)
  arc A257 (-239.0313, 59.675) -> (-238.5313, 60.175) centre (-239.0313, 60.175) ccw
  arc A258 (-240.0312, 60.175) -> (-239.5312, 59.675) centre (-239.5312, 60.175) ccw
  arc A259 (-238.5312, 73.175) -> (-239.0313, 73.675) centre (-239.0312, 73.175) ccw
  arc A260 (-239.5312, 73.675) -> (-240.0312, 73.175) centre (-239.5312, 73.175) ccw
  line L272 (-260.5312, 59.675) -> (-261.0312, 59.675)
  line L273 (-260.5313, 73.675) -> (-261.0312, 73.675)
  line L274 (-269.725, 59.675) -> (-282.725, 59.675)
  line L275 (-275.4942, 73.675) -> (-282.725, 73.675)
  line L276 (-269.225, 60.175) -> (-269.225, 60.175)
  line L277 (-283.225, 60.175) -> (-283.225, 73.175)
  arc A261 (-269.725, 59.675) -> (-269.225, 60.175) centre (-269.725, 60.175) ccw
  arc A262 (-283.225, 60.175) -> (-282.725, 59.675) centre (-282.725, 60.175) ccw
  arc A263 (-282.725, 73.675) -> (-283.225, 73.175) centre (-282.725, 73.175) ccw
  line L278 (-31.6, 78.725) -> (-44.6, 78.725)
  line L279 (-31.6, 92.725) -> (-44.6, 92.725)
  line L280 (-31.1, 79.225) -> (-31.1, 92.225)
  line L281 (-45.1, 79.225) -> (-45.1, 92.225)
  arc A264 (-31.6, 78.725) -> (-31.1, 79.225) centre (-31.6, 79.225) ccw
  arc A265 (-45.1, 79.225) -> (-44.6, 78.725) centre (-44.6, 79.225) ccw
  arc A266 (-31.1, 92.225) -> (-31.6, 92.725) centre (-31.6, 92.225) ccw
  arc A267 (-44.6, 92.725) -> (-45.1, 92.225) centre (-44.6, 92.225) ccw
  line L282 (-55.4125, 78.725) -> (-68.4125, 78.725)
  line L283 (-55.4125, 92.725) -> (-68.4125, 92.725)
  line L284 (-54.9125, 79.225) -> (-54.9125, 92.225)
  line L285 (-68.9125, 79.225) -> (-68.9125, 92.225)
  arc A268 (-55.4125, 78.725) -> (-54.9125, 79.225) centre (-55.4125, 79.225) ccw
  arc A269 (-68.9125, 79.225) -> (-68.4125, 78.725) centre (-68.4125, 79.225) ccw
  arc A270 (-54.9125, 92.225) -> (-55.4125, 92.725) centre (-55.4125, 92.225) ccw
  arc A271 (-68.4125, 92.725) -> (-68.9125, 92.225) centre (-68.4125, 92.225) ccw
  line L286 (-50.9125, 78.725) -> (-51.4125, 78.725)
  line L287 (-50.9125, 92.725) -> (-51.4125, 92.725)
  line L288 (-50.4125, 79.225) -> (-50.4125, 92.225)
  line L289 (-51.9125, 79.225) -> (-51.9125, 92.225)
  arc A272 (-50.9125, 78.725) -> (-50.4125, 79.225) centre (-50.9125, 79.225) ccw
  arc A273 (-51.9125, 79.225) -> (-51.4125, 78.725) centre (-51.4125, 79.225) ccw
  arc A274 (-50.4125, 92.225) -> (-50.9125, 92.725) centre (-50.9125, 92.225) ccw
  arc A275 (-51.4125, 92.725) -> (-51.9125, 92.225) centre (-51.4125, 92.225) ccw
  line L290 (-72.4125, 78.725) -> (-72.9125, 78.725)
  line L291 (-72.4125, 92.725) -> (-72.9125, 92.725)
  line L292 (-71.9125, 79.225) -> (-71.9125, 92.225)
  line L293 (-73.4125, 79.225) -> (-73.4125, 92.225)
  arc A276 (-72.4125, 78.725) -> (-71.9125, 79.225) centre (-72.4125, 79.225) ccw
  arc A277 (-73.4125, 79.225) -> (-72.9125, 78.725) centre (-72.9125, 79.225) ccw
  arc A278 (-71.9125, 92.225) -> (-72.4125, 92.725) centre (-72.4125, 92.225) ccw
  arc A279 (-72.9125, 92.725) -> (-73.4125, 92.225) centre (-72.9125, 92.225) ccw
  line L294 (-126.85, 78.725) -> (-139.85, 78.725)
  line L295 (-126.85, 92.725) -> (-139.85, 92.725)
  line L296 (-126.35, 79.225) -> (-126.35, 92.225)
  line L297 (-140.35, 79.225) -> (-140.35, 92.225)
  arc A280 (-126.85, 78.725) -> (-126.35, 79.225) centre (-126.85, 79.225) ccw
  arc A281 (-140.35, 79.225) -> (-139.85, 78.725) centre (-139.85, 79.225) ccw
  arc A282 (-126.35, 92.225) -> (-126.85, 92.725) centre (-126.85, 92.225) ccw
  arc A283 (-139.85, 92.725) -> (-140.35, 92.225) centre (-139.85, 92.225) ccw
  line L298 (-82.725, 79.725) -> (-88.725, 79.725)
  line L299 (-82.725, 94.725) -> (-88.725, 94.725)
  line L300 (-82.225, 80.225) -> (-82.225, 94.225)
  line L301 (-89.225, 80.225) -> (-89.225, 94.225)
  arc A284 (-82.725, 79.725) -> (-82.225, 80.225) centre (-82.725, 80.225) ccw
  arc A285 (-89.225, 80.225) -> (-88.725, 79.725) centre (-88.725, 80.225) ccw
  arc A286 (-82.225, 94.225) -> (-82.725, 94.725) centre (-82.725, 94.225) ccw
  arc A287 (-88.725, 94.725) -> (-89.225, 94.225) centre (-88.725, 94.225) ccw
  line L302 (-177.975, 79.725) -> (-183.975, 79.725)
  line L303 (-177.975, 94.725) -> (-183.975, 94.725)
  line L304 (-177.475, 80.225) -> (-177.475, 94.225)
  line L305 (-184.475, 80.225) -> (-184.475, 94.225)
  arc A288 (-177.975, 79.725) -> (-177.475, 80.225) centre (-177.975, 80.225) ccw
  arc A289 (-184.475, 80.225) -> (-183.975, 79.725) centre (-183.975, 80.225) ccw
  arc A290 (-177.475, 94.225) -> (-177.975, 94.725) centre (-177.975, 94.225) ccw
  arc A291 (-183.975, 94.725) -> (-184.475, 94.225) centre (-183.975, 94.225) ccw
  line L306 (-198.2875, 78.725) -> (-211.2875, 78.725)
  line L307 (-198.2875, 92.725) -> (-211.2875, 92.725)
  line L308 (-197.7875, 79.225) -> (-197.7875, 92.225)
  line L309 (-211.7875, 79.225) -> (-211.7875, 92.225)
  arc A292 (-198.2875, 78.725) -> (-197.7875, 79.225) centre (-198.2875, 79.225) ccw
  arc A293 (-211.7875, 79.225) -> (-211.2875, 78.725) centre (-211.2875, 79.225) ccw
  arc A294 (-197.7875, 92.225) -> (-198.2875, 92.725) centre (-198.2875, 92.225) ccw
  arc A295 (-211.2875, 92.725) -> (-211.7875, 92.225) centre (-211.2875, 92.225) ccw
  line L310 (-193.7875, 78.725) -> (-194.2875, 78.725)
  line L311 (-193.7875, 92.725) -> (-194.2875, 92.725)
  line L312 (-193.2875, 79.225) -> (-193.2875, 92.225)
  line L313 (-194.7875, 79.225) -> (-194.7875, 92.225)
  arc A296 (-193.7875, 78.725) -> (-193.2875, 79.225) centre (-193.7875, 79.225) ccw
  arc A297 (-194.7875, 79.225) -> (-194.2875, 78.725) centre (-194.2875, 79.225) ccw
  arc A298 (-193.2875, 92.225) -> (-193.7875, 92.725) centre (-193.7875, 92.225) ccw
  arc A299 (-194.2875, 92.725) -> (-194.7875, 92.225) centre (-194.2875, 92.225) ccw
  line L314 (-215.2875, 78.725) -> (-215.7875, 78.725)
  line L315 (-215.2875, 92.725) -> (-215.7875, 92.725)
  line L316 (-214.7875, 79.225) -> (-214.7875, 92.225)
  line L317 (-216.2875, 79.225) -> (-216.2875, 92.225)
  arc A300 (-215.2875, 78.725) -> (-214.7875, 79.225) centre (-215.2875, 79.225) ccw
  arc A301 (-216.2875, 79.225) -> (-215.7875, 78.725) centre (-215.7875, 79.225) ccw
  arc A302 (-214.7875, 92.225) -> (-215.2875, 92.725) centre (-215.2875, 92.225) ccw
  arc A303 (-215.7875, 92.725) -> (-216.2875, 92.225) centre (-215.7875, 92.225) ccw
  line L318 (-222.1, 78.725) -> (-235.1, 78.725)
  line L319 (-222.1, 92.725) -> (-235.1, 92.725)
  line L320 (-221.6, 79.225) -> (-221.6, 92.225)
  line L321 (-235.6, 79.225) -> (-235.6, 92.225)
  arc A304 (-222.1, 78.725) -> (-221.6, 79.225) centre (-222.1, 79.225) ccw
  arc A305 (-235.6, 79.225) -> (-235.1, 78.725) centre (-235.1, 79.225) ccw
  arc A306 (-221.6, 92.225) -> (-222.1, 92.725) centre (-222.1, 92.225) ccw
  arc A307 (-235.1, 92.725) -> (-235.6, 92.225) centre (-235.1, 92.225) ccw
  line L322 (0, 95.25) -> (-285.75, 95.25)
  line L323 (0, 0) -> (-285.75, 0)
  line L324 (0, 95.25) -> (0, 0)
  line L325 (-285.75, 95.25) -> (-285.75, 0)
  line L326 (-243.5313, 73.675) -> (-243.6182, 73.675)
  line L327 (-251.6182, 73.675) -> (-256.5312, 73.675)
  line L328 (-250.675, 16.525) -> (-250.762, 16.525)
  line L329 (-258.762, 16.525) -> (-263.675, 16.525)
  line L330 (-269.725, 16.525) -> (-274.638, 16.525)
  line L331 (-282.638, 16.525) -> (-282.725, 16.525)
  arc A308 (-251.262, 17.025) -> (-250.762, 16.525) centre (-250.762, 17.025) ccw
  arc A309 (-258.762, 16.525) -> (-258.262, 17.025) centre (-258.762, 17.025) ccw
  arc A310 (-275.138, 17.025) -> (-274.638, 16.525) centre (-274.638, 17.025) ccw
  arc A311 (-282.638, 16.525) -> (-282.138, 17.025) centre (-282.638, 17.025) ccw
  arc A312 (-268.725, 60.675) -> (-269.225, 60.175) centre (-268.725, 60.175) ccw
  arc A313 (-275.4942, 73.675) -> (-274.9942, 74.175) centre (-275.4942, 74.175) ccw
  arc A314 (-251.6182, 73.675) -> (-251.1182, 74.175) centre (-251.6182, 74.175) ccw
  arc A315 (-244.1182, 74.175) -> (-243.6182, 73.675) centre (-243.6182, 74.175) ccw
  point P0 (-282.725, 16.525)
  point P1 (-243.5313, 73.675)
  point P2 (-269.225, 60.175)
  dimension "d0" = 0.5
  constraints: 664 end point, 632 point on circle, 316 centre point, 16 tangent, 7 equal radius
  measures "d0" radius of A308
extrude "Extrusion1" add sketch "Sketch1" along normal blind 1.5
body "Solid1"
